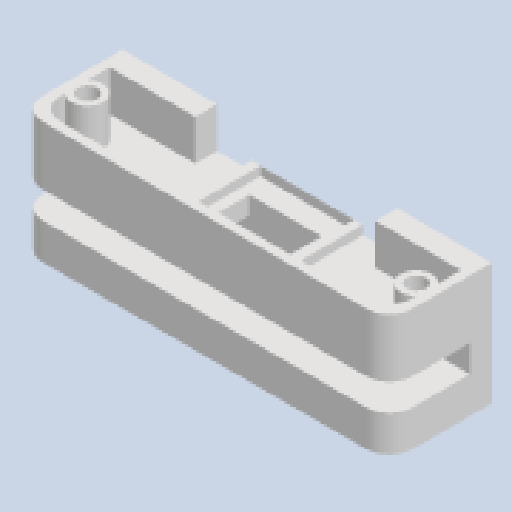
# Autodesk Inventor part: basepcb
Saved by Autodesk Inventor 2026.2 (Build 302298000, 298)
## iProperties
Created: 2026-04-10
Part Number: basepcb
Material: Generic
Document SubType Name: Modeling
Designer: Fork
Density: 1 g/cm^3
Appearance: Default
Author: Fork
Autodesk Inventor part; units mm, degrees
ref_plane "YZ Plane" through (0, 0, 0) normal (1, 0, 0) x (0, 1, 0)
ref_plane "XZ Plane" through (0, 0, 0) normal (0, 1, 0) x (-1, 0, 0)
ref_plane "XY Plane" through (0, 0, 0) normal (0, 0, 1) x (1, 0, 0)
sketch "Sketch1" plane through (0, 0, 0) normal (0, 1, 0) x (-1, 0, 0)
  line L0 (-33.5, 62.1) -> (33.5, 62.1)
  line L1 (33.5, 62.1) -> (33.5, -62.1)
  line L2 (33.5, -62.1) -> (-33.5, -62.1)
  line L3 (-33.5, -62.1) -> (-33.5, 62.1)
  line L4 (-33.5, 62.1) -> (33.5, -62.1) construction
  line L5 (33.5, 62.1) -> (-33.5, -62.1) construction
  line L6 (30.5, -59.1) -> (30.5, 59.1)
  line L7 (30.5, 59.1) -> (-30.5, 59.1)
  line L8 (-30.5, 59.1) -> (-30.5, -59.1)
  line L9 (-30.5, -59.1) -> (30.5, -59.1)
  circle A0 centre (30.5, 59.1) radius 2.25
  circle A1 centre (-30.5, 59.1) radius 2.25
  circle A2 centre (-30.5, -59.1) radius 2.25
  circle A3 centre (30.5, -59.1) radius 2.25
  line L10 (-41, 71) -> (41, 71)
  line L11 (41, 71) -> (41, -71)
  line L12 (41, -71) -> (-41, -71)
  line L13 (-41, -71) -> (-41, 71)
  line L14 (-41, 71) -> (41, -71) construction
  line L15 (41, 71) -> (-41, -71) construction
  line L16 (12.75, 87.6) -> (-7.75, 87.6)
  line L17 (-7.75, 87.6) -> (-7.75, 67.1)
  line L18 (-7.75, 67.1) -> (12.75, 67.1)
  line L19 (12.75, 67.1) -> (12.75, 87.6)
  line L20 (12.75, 87.6) -> (-7.75, 67.1) construction
  line L21 (-7.75, 87.6) -> (12.75, 67.1) construction
  line L22 (41, 71) -> (-41, 71)
  line L23 (-41, 71) -> (-41, 92)
  line L24 (-41, 92) -> (41, 92)
  line L25 (41, 92) -> (41, 71)
  point P0 (0, 0)
  point P1 (2.5, 77.35)
  point P2 (12.75, 77.35)
  point P3 (-41, 71)
  dimension "d0" = 67
  dimension "d1" = 124.2
  dimension "d2" = 3
  dimension "d3" = 4.5
  dimension "d4" = 4.5
  dimension "d5" = 4.5
  dimension "d6" = 4.5
  dimension "d9" = 82
  dimension "d10" = 142
  dimension "d27" = 20.5
  dimension "d28" = 20.5
  dimension "d29" = 5
  dimension "d30" = 28.25
  dimension "d31" = 82
  dimension "d32" = 21
  constraints: 52 end point, 10 parallel, 7 midpoint, 5 perpendicular, 4 centre point, 4 coincident, 4 horizontal, 3 other
  measures "d0" distance of L1.end L2.end
  measures "d1" distance of L0.end L1.end
  measures "d2" distance between parallel lines of L1 L6
  measures "d3" diameter of A0
  measures "d4" diameter of A1
  measures "d5" diameter of A2
  measures "d6" diameter of A3
  measures "d9" distance of L11.end L12.end
  measures "d10" distance of L10.end L11.end
  measures "d27" distance of L18.end L17.end
  measures "d28" distance of L17.end L16.end
  measures "d29" distance between parallel lines of L0 L18
  measures "d30" distance from line of L11 point (12.75, 77.35)
  measures "d31" distance of L23.end L24.end
  measures "d32" distance of L22.end L23.end
extrude "Extrusion1" add sketch "Sketch1" along normal blind 2 contours L0 L1 L2 L3 | L9 A3 L6 | L6 A3 L9 | A3 L9 A2 L8 A1 L7 A0 L6 | A0 L7 L6 | L6 L7 A0 | A2 L8 L9 | L9 L8 A2 | A1 L8 L7 | L7 L8 A1 | L23 L24 L25 L10 L19 L16 L17 | L10 L17 L18 L19 L11 L12 L13 | L17 L16 L19 L10 | L10 L19 L18 L17
sketch "Sketch3" plane through (0, 2, 0) normal (0, 1, 0) x (1, 0, 0)
  line L0 (33.5, -62.1) -> (-33.5, -62.1)
  line L1 (-33.5, -62.1) -> (-33.5, 62.1)
  line L2 (-33.5, 62.1) -> (33.5, 62.1)
  line L3 (33.5, 62.1) -> (33.5, -62.1)
  line L4 (33.5, -62.1) -> (-33.5, 62.1) construction
  line L5 (-33.5, -62.1) -> (33.5, 62.1) construction
  line L6 (-30.5, -59.1) -> (30.5, -59.1)
  line L7 (30.5, -59.1) -> (30.5, 59.1)
  line L8 (30.5, 59.1) -> (-30.5, 59.1)
  line L9 (-30.5, 59.1) -> (-30.5, -59.1)
  circle A0 centre (-30.5, -59.1) radius 2.25
  circle A1 centre (-30.5, 59.1) radius 2.25
  circle A2 centre (30.5, -59.1) radius 2.25
  circle A3 centre (30.5, 59.1) radius 2.25
  circle A4 centre (-30.5, -59.1) radius 5.25
  circle A5 centre (30.5, -59.1) radius 5.25
  circle A6 centre (-30.5, 59.1) radius 5.25
  circle A7 centre (30.5, 59.1) radius 5.25
  point P0 (0, 0)
  dimension "d11" = 67
  dimension "d12" = 124.2
  dimension "d13" = 3
  dimension "d14" = 4.5
  dimension "d15" = 4.5
  dimension "d16" = 4.5
  dimension "d17" = 4.5
  dimension "d18" = 3
  dimension "d19" = 3
  dimension "d20" = 3
  dimension "d21" = 3
  constraints: 20 end point, 8 centre point, 4 coincident, 4 parallel, 2 midpoint, 2 perpendicular, 1 horizontal, 3 other
  measures "d11" distance of L1.end L2.end
  measures "d12" distance of L0.end L1.end
  measures "d13" distance between parallel lines of L0 L6
  measures "d14" diameter of A0
  measures "d15" diameter of A1
  measures "d16" diameter of A2
  measures "d17" diameter of A3
  measures "d18" radial gap between concentric circles of A0 A4
  measures "d19" radial gap between concentric circles of A2 A5
  measures "d20" radial gap between concentric circles of A1 A6
  measures "d21" radial gap between concentric circles of A3 A7
extrude "Extrusion2" add sketch "Sketch3" along normal blind 15 contours L3 A5 L0 | L0 A5 L6 A2 L7 L3 | A4 L1 L0 | L0 L1 A4 L9 A0 L6 | A5 L7 A2 L6 | A7 L7 A3 L8 L2 L3 | L3 L2 A7 | L6 A0 L9 A4 | A7 L8 A3 L7 | A6 L2 L1 | L1 L2 A6 L8 A1 L9 | L9 A1 L8 A6
sketch "Sketch5" plane through (0, 2, 0) normal (0, 1, 0) x (1, 0, 0)
  line L0 (41, 71) -> (-41, 71) projected
  line L1 (-41, 71) -> (-41, -92) projected
  line L2 (41, 71) -> (-41, 71)
  line L3 (-41, 71) -> (-41, -92)
  line L4 (41, -92) -> (41, 71) projected
  line L5 (-41, -66.1) -> (-41, 71)
  circle A0 centre (-30.5, -59.1) radius 5.25 projected
  line L6 (-41, 71) -> (41, 71)
  line L7 (41, 71) -> (41, -71.1)
  line L8 (41, -71.1) -> (-41, -71.1)
  line L9 (-41, -71.1) -> (-41, 71)
  line L10 (-39, -69.1) -> (39, -69.1)
  line L11 (39, -69.1) -> (39, 69)
  line L12 (39, 69) -> (-39, 69)
  line L13 (-39, 69) -> (-39, -69.1)
  line L14 (-20, -69.1) -> (20, -69.1)
  line L15 (20, -69.1) -> (20, -71.1)
  line L16 (20, -71.1) -> (-20, -71.1)
  line L17 (-20, -71.1) -> (-20, -69.1)
  point P0 (0, 0)
  point P1 (-20, -70.1)
  point P2 (0, -69.1)
  point P3 (-41, -71.1)
  dimension "d107" = 12
  dimension "d108" = 2
  dimension "d109" = 2
  dimension "d110" = 2
  dimension "d111" = 2
  dimension "d112" = 40
  dimension "d113" = 2
  dimension "d114" = 20
  constraints: 30 end point, 6 parallel, 4 horizontal, 4 perpendicular, 2 midpoint, 2 point on line
  measures "d107" distance from line of L8 A0.centre
  measures "d108" distance between parallel lines of L1 L13
  measures "d109" distance between parallel lines of L8 L10
  measures "d110" distance between parallel lines of L4 L11
  measures "d111" distance between parallel lines of L0 L12
  measures "d112" distance of L15.end L16.end
  measures "d113" distance of L14.end L15.end
  measures "d114" horizontal distance of point (-20, -70.1) point (0, -69.1)
extrude "Extrusion4" add sketch "Sketch5" along normal blind 25 contours L4 L8 L15 L10 L11 L12 L13 L17 L1 L0
sketch "Sketch7" plane through (0, 2, 0) normal (0, 1, 0) x (1, 0, 0)
  circle A0 centre (-36, 66) radius 2.1
  circle A1 centre (-36, 66) radius 4
  circle A2 centre (36, 66) radius 2.1
  circle A3 centre (-36, -66.1) radius 2.1
  circle A4 centre (36, -66.1) radius 2.1
  circle A5 centre (36, 66) radius 4
  circle A6 centre (36, -66.1) radius 4
  circle A7 centre (-36, -66.1) radius 4
  line L0 (-39, -69.1) -> (-39, 69) projected
  line L1 (-39, 69) -> (39, 69) projected
  line L2 (-20, -69.1) -> (-39, -69.1) projected
  line L3 (39, 69) -> (39, -69.1) projected
  line L4 (39, -69.1) -> (20, -69.1) projected
  point P0 (0, 0)
  dimension "d36" = 4.2
  dimension "d39" = 8
  dimension "d44" = 4.2
  dimension "d45" = 4.2
  dimension "d46" = 4.2
  dimension "d53" = 8
  dimension "d54" = 8
  dimension "d55" = 8
  dimension "d115" = 3
  dimension "d116" = 3
  dimension "d117" = 3
  dimension "d118" = 3
  dimension "d119" = 3
  dimension "d121" = 3
  dimension "d122" = 3
  dimension "d123" = 3
  constraints: 8 centre point, 4 coincident
  measures "d36" diameter of A0
  measures "d39" diameter of A1
  measures "d44" diameter of A2
  measures "d45" diameter of A3
  measures "d46" diameter of A4
  measures "d53" diameter of A5
  measures "d54" diameter of A6
  measures "d55" diameter of A7
  measures "d115" distance from line of L0 A0.centre
  measures "d116" distance from line of L1 A0.centre
  measures "d117" distance from line of L2 A7.centre
  measures "d118" distance from line of L0 A7.centre
  measures "d119" distance from line of L3 A6.centre
  measures "d121" distance from line of L3 A5.centre
  measures "d122" distance from line of L1 A2.centre
  measures "d123" distance from line of L4 A4.centre
extrude "Extrusion5" add sketch "Sketch7" along normal up to surface (25 mm away) contours A1 L0 L1 | L1 A1 | A1 L0 | A5 L3 | L3 A5 L1 | L1 A5 | A6 L3 | L3 A6 L4 | L4 A6 | A7 L2 L0 | L0 A7 | A7 L2 picked at (-35.9156, 68.6949) picked at (36.0844, 68.6949) picked at (36.0844, -68.7949) picked at (-36.0844, -68.7949)
sketch "Sketch8" plane through (0, 2, 0) normal (0, 1, 0) x (1, 0, 0)
  line L0 (41, -92) -> (41, -71.1) projected
  line L1 (-41, -92) -> (41, -92)
  line L2 (41, -92) -> (41, -71.1)
  line L3 (41, -71.1) -> (-41, -71.1)
  line L4 (-41, -71.1) -> (-41, -92)
  point P0 (0, 0)
  point P1 (37.4215, -69.1)
  constraints: 8 end point, 2 parallel, 1 horizontal, 1 perpendicular
extrude "Extrusion6" add sketch "Sketch8" along normal blind 8
sketch "Sketch18" plane through (20, 27, 71.1) normal (0, 0, 1) x (1, 0, 0)
  line L0 (-61, -27) -> (-61, 0) projected
  line L1 (21, -27) -> (21, 0) projected
  line L2 (-61, 0) -> (21, 0)
  line L3 (21, 0) -> (21, -13)
  line L4 (21, -13) -> (-61, -13)
  line L5 (-61, -13) -> (-61, 0)
  line L6 (-61, -17) -> (21, -17) projected
  line L7 (-61, -13) -> (21, -13)
  line L8 (21, -13) -> (21, -3)
  line L9 (21, -3) -> (-61, -3)
  line L10 (-61, -3) -> (-61, -13)
  point P0 (-20, -27)
  point P1 (21, -3)
  dimension "d124" = 4
  dimension "d125" = 10
  constraints: 16 end point, 4 parallel, 2 horizontal, 2 perpendicular, 2 point on line
  measures "d124" distance between parallel lines of L4 L6
  measures "d125" distance of L8.end L7.end
extrude "Extrusion16" add sketch "Sketch18" along normal up to surface (20.9 mm away) contours L0 L9 L1 L4
sketch "Sketch19" plane through (-20, 24, 71.1) normal (0, 1, 0) x (1, 0, 0)
  line L0 (-21, 142.1) -> (-21, -20.9) projected
  line L1 (40, 0) -> (61, 0) projected
  line L2 (-21, -20.9) -> (61, -20.9)
  line L3 (61, -20.9) -> (61, 0)
  line L4 (61, 0) -> (-21, 0)
  line L5 (-21, 0) -> (-21, -20.9)
  line L6 (-19, -2) -> (59, -2)
  line L7 (59, -2) -> (59, -18.9)
  line L8 (59, -18.9) -> (-19, -18.9)
  line L9 (-19, -18.9) -> (-19, -2)
  line L10 (0, 0) -> (0, -2)
  line L11 (40, 0) -> (40, -2)
  point P0 (20, 71.1)
  dimension "d128" = 2
  constraints: 20 end point, 4 parallel, 4 perpendicular, 2 point on line, 1 horizontal, 3 other
  measures "d128" distance between parallel lines of L4 L6
extrude "Extrusion17" cut sketch "Sketch19" against normal blind 6 contours L4 L11 L6 L10 | L6 L7 L8 L9
sketch "Sketch20" plane through (-20, 18, 71.1) normal (0, 1, 0) x (1, 0, 0)
  line L0 (59, -18.9) -> (-19, -18.9) projected
  line L1 (20, -18.9) -> (20, 0)
  line L2 (0, 0) -> (40, 0) projected
  circle A0 centre (12.1, -15.9) radius 1.75
  circle A1 centre (27.9, -15.9) radius 1.75
  point P0 (20, 71.1)
  dimension "d131" = 3.5
  dimension "d132" = 3.5
  dimension "d133" = 15.8
  dimension "d134" = 7.9
  dimension "d135" = 3
  dimension "d136" = 3
  constraints: 2 centre point, 2 end point, 2 midpoint
  measures "d131" diameter of A0
  measures "d132" diameter of A1
  measures "d133" distance of A1.centre A0.centre
  measures "d134" distance from line of A0.centre L1
  measures "d135" distance from line of L0 A0.centre
  measures "d136" distance from line of L0 A1.centre
sketch "Sketch21" plane through (0, 2, 0) normal (0, 1, 0) x (1, 0, 0)
  line L0 (20, -69.1) -> (20, -71.1) projected
  line L1 (-20, -71.1) -> (20, -71.1) projected
  line L2 (20, -69.1) -> (-20, -69.1)
  line L3 (-20, -69.1) -> (-20, -71.1)
  line L4 (-20, -71.1) -> (20, -71.1)
  line L5 (20, -71.1) -> (20, -69.1)
  point P0 (0, 0)
  constraints: 8 end point, 2 parallel, 1 horizontal, 1 perpendicular
extrude "Extrusion18" add sketch "Sketch21" along normal up to surface (16 mm away)
extrude "Extrusion19" cut sketch "Sketch20" against normal blind 4
sketch "Sketch22" plane through (-20, 18, 71.1) normal (0, 1, 0) x (1, 0, 0)
  line L0 (30.35, 1.8) -> (9.65, 1.8)
  line L1 (9.65, 1.8) -> (9.65, -18.9)
  line L2 (9.65, -18.9) -> (30.35, -18.9)
  line L3 (30.35, -18.9) -> (30.35, 1.8)
  line L4 (30.35, 1.8) -> (9.65, -18.9) construction
  line L5 (9.65, 1.8) -> (30.35, -18.9) construction
  line L6 (40, 2) -> (0, 2) projected
  line L7 (20, 2) -> (20, -18.9)
  line L8 (59, -18.9) -> (-19, -18.9) projected
  line L9 (59, -18.9) -> (-19, -18.9) projected
  line L10 (32.35, 3.8) -> (7.65, 3.8)
  line L11 (7.65, 3.8) -> (7.65, -20.9)
  line L12 (7.65, -20.9) -> (32.35, -20.9)
  line L13 (32.35, -20.9) -> (32.35, 3.8)
  point P0 (20, 71.1)
  point P1 (20, -8.55)
  point P2 (20, -18.9)
  point P3 (32.35, -18.9)
  point P4 (32.35, 2)
  point P5 (7.65, 2)
  point P6 (7.65, -18.9)
  point P7 (9.65, -18.9)
  point P8 (30.35, -18.9)
  dimension "d141" = 20.7
  dimension "d142" = 20.7
  dimension "d143" = 0
  dimension "d144" = 0
  dimension "d145" = 2
  constraints: 22 end point, 5 midpoint, 4 parallel, 2 perpendicular, 1 horizontal, 3 other
  measures "d141" distance of L2.end L1.end
  measures "d142" distance of L0.end L1.end
  measures "d143" horizontal distance of point (20, -18.9) point (20, -8.55)
  measures "d144" distance between parallel lines of L8 L2
  measures "d145" distance between parallel lines of L3 L13
extrude "Extrusion20" add sketch "Sketch22" along normal blind 2 contours L0 L7 L6 L13 L8 L3 | L0 L1 L8 L11 L6 L7
sketch "Sketch23" plane through (-20, 18, 71.1) normal (0, 1, 0) x (1, 0, 0)
  line L0 (-13.3542, 2) -> (53.3542, 2) projected
  line L1 (20, 2) -> (20, -18.9)
  line L2 (30.35, -18.9) -> (9.65, -18.9) projected
  line L3 (28, -13.9) -> (12, -13.9)
  line L4 (12, -13.9) -> (12, -1.9)
  line L5 (12, -1.9) -> (28, -1.9)
  line L6 (28, -1.9) -> (28, -13.9)
  circle A0 centre (27.9, -15.9) radius 1.75 projected
  point P0 (20, 71.1)
  point P1 (28, -7.9)
  point P2 (20, -13.9)
  dimension "d148" = 8
  dimension "d149" = 8
  dimension "d150" = 2
  dimension "d151" = 12
  constraints: 10 end point, 4 midpoint, 2 parallel, 1 horizontal, 1 perpendicular
  measures "d148" distance from line of point (28, -7.9) L1
  measures "d149" distance between parallel lines of L4 L1
  measures "d150" vertical distance of A0.centre point (20, -13.9)
  measures "d151" distance between parallel lines of L3 L5
extrude "Extrusion21" cut sketch "Sketch23" against normal blind 4 contours L5 L6 L3 L1 | L1 L3 L4 L5
sketch "Sketch24" plane through (41, 0, -71) normal (0, 0, -1) x (-1, 0, 0)
  line L0 (34.3117, 23.869) -> (40.9117, 23.869) projected
  arc A0 (42.2117, 22.569) -> (40.9117, 23.869) centre (40.9117, 22.569) ccw projected
  line L1 (42.2117, 22.569) -> (42.2117, 21.9283) projected
  line L2 (37.3524, 20.6283) -> (34.3117, 20.6283) projected
  arc A1 (33.0117, 21.9283) -> (34.3117, 20.6283) centre (34.3117, 21.9283) ccw projected
  line L3 (33.0117, 22.3283) -> (33.0117, 21.9283) projected
  arc A2 (34.3117, 23.869) -> (33.0117, 22.569) centre (34.3117, 22.569) ccw projected
  line L4 (33.0117, 21.9283) -> (33.0117, 22.569) projected
  arc A3 (40.9117, 20.6283) -> (42.2117, 21.9283) centre (40.9117, 21.9283) ccw projected
  line L5 (40.9117, 20.6283) -> (37.371, 20.6283) projected
  line L6 (37.371, 20.6283) -> (37.3524, 20.6283) projected
  line L7 (40.9117, 24.169) -> (34.3117, 24.169)
  arc A4 (34.3117, 24.169) -> (32.7117, 22.569) centre (34.3117, 22.569) ccw
  line L8 (32.7117, 22.569) -> (32.7117, 21.9283)
  arc A5 (32.7117, 21.9283) -> (34.3117, 20.3283) centre (34.3117, 21.9283) ccw
  line L9 (34.3117, 20.3283) -> (37.3524, 20.3283)
  line L10 (37.3524, 20.3283) -> (37.371, 20.3283)
  line L11 (37.371, 20.3283) -> (40.9117, 20.3283)
  arc A6 (40.9117, 20.3283) -> (42.5117, 21.9283) centre (40.9117, 21.9283) ccw
  line L12 (42.5117, 21.9283) -> (42.5117, 22.569)
  arc A7 (42.5117, 22.569) -> (40.9117, 24.169) centre (40.9117, 22.569) ccw
  point P0 (41, 0)
  dimension "d154" = 0.3
  constraints: 12 end point, 8 point on circle, 4 centre point, 9 other
  measures "d154" radial gap between concentric circles of A0 A7
extrude "Extrusion22" cut sketch "Sketch24" against normal blind 2 contours L0 A0 L1 A3 L5 L6 L2 A1 L3 L4 A2 | A7 L12 A6 L11 L10 L9 A5 L8 A4 L7
sketch "Sketch25" plane through (-33.3542, 2, -69) normal (0, 0, 1) x (1, 0, 0)
  line L0 (41.6426, 20.569) -> (41.6426, 19.9283) projected
  arc A0 (40.0426, 18.3283) -> (41.6426, 19.9283) centre (40.0426, 19.9283) ccw projected
  line L1 (40.0426, 18.3283) -> (33.4426, 18.3283) projected
  arc A1 (31.8426, 19.9283) -> (33.4426, 18.3283) centre (33.4426, 19.9283) ccw projected
  line L2 (31.8426, 19.9283) -> (31.8426, 20.569) projected
  arc A2 (33.4426, 22.169) -> (31.8426, 20.569) centre (33.4426, 20.569) ccw projected
  line L3 (33.4426, 22.169) -> (40.0426, 22.169) projected
  arc A3 (41.6426, 20.569) -> (40.0426, 22.169) centre (40.0426, 20.569) ccw projected
  line L4 (66.7085, 0) -> (66.7085, 25) projected
  line L5 (0, 25) -> (66.7085, 25) projected
  line L6 (0, 25) -> (0, 0) projected
  line L7 (66.7085, 0) -> (0, 0) projected
  line L8 (30.8426, 20.569) -> (30.8426, 19.9283)
  arc A4 (30.8426, 19.9283) -> (33.4426, 17.3283) centre (33.4426, 19.9283) ccw
  line L9 (33.4426, 17.3283) -> (40.0426, 17.3283)
  arc A5 (40.0426, 17.3283) -> (42.6426, 19.9283) centre (40.0426, 19.9283) ccw
  line L10 (42.6426, 19.9283) -> (42.6426, 20.569)
  arc A6 (42.6426, 20.569) -> (40.0426, 23.169) centre (40.0426, 20.569) ccw
  line L11 (40.0426, 23.169) -> (33.4426, 23.169)
  arc A7 (33.4426, 23.169) -> (30.8426, 20.569) centre (33.4426, 20.569) ccw
  point P0 (33.3542, -2)
  dimension "d157" = 1
  constraints: 8 end point, 8 point on circle, 4 centre point, 7 other
  measures "d157" radial gap between concentric circles of A2 A7
extrude "Extrusion23" add sketch "Sketch25" along normal blind 1 contours A7 L11 A6 L10 A5 L9 A4 L8
sketch "Sketch26" plane through (41, 0, -71) normal (0, 0, -1) x (-1, 0, 0)
  line L0 (28.8617, 19.1283) -> (46.3617, 19.1283)
  line L1 (46.3617, 19.1283) -> (46.3617, 17.1283)
  line L2 (46.3617, 17.1283) -> (28.8617, 17.1283)
  line L3 (28.8617, 17.1283) -> (28.8617, 19.1283)
  line L4 (34.3117, 19.3283) -> (40.9117, 19.3283) projected
  point P0 (41, 0)
  point P1 (37.6117, 19.3283)
  point P2 (28.8617, 18.1283)
  dimension "d160" = 0.2
  dimension "d161" = 17.5
  dimension "d162" = 8.75
  dimension "d163" = 2
  constraints: 8 end point, 2 midpoint, 2 parallel, 1 horizontal, 1 perpendicular
  measures "d160" distance between parallel lines of L4 L0
  measures "d161" distance of L1.end L2.end
  measures "d162" horizontal distance of point (37.612, 19.328) point (28.862, 18.128)
  measures "d163" distance of L0.end L1.end
extrude "Extrusion24" add sketch "Sketch26" against normal blind 8
fillet "Fillet1" radius 5 6 edges at (-41, 13.5, -71) (41, 13.5, -71) (-41, 5, 92) (-41, 19, 92) (41, 5, 92) (41, 19, 92)
sketch "Sketch27" plane through (-41, 10, 71.1) normal (-1, 0, 0) x (0, 0, 1)
  line L0 (-117.1, 11) -> (-109.6, 11)
  line L1 (-109.6, 11) -> (-109.6, 6)
  line L2 (-109.6, 6) -> (-117.1, 6)
  line L3 (-117.1, 6) -> (-117.1, 11)
  line L4 (-142.1, 17) -> (-142.1, -10) projected
  line L5 (-137.1, 17) -> (0, 17) projected
  point P0 (-71.1, -10)
  point P1 (-117.1, 8.5)
  dimension "d167" = 7.5
  dimension "d168" = 5
  dimension "d169" = 25
  dimension "d170" = 6
  constraints: 8 end point, 2 parallel, 1 horizontal, 1 midpoint, 1 perpendicular
  measures "d167" distance of L1.end L2.end
  measures "d168" distance of L0.end L1.end
  measures "d169" distance from line of L4 point (-117.1, 8.5)
  measures "d170" distance between parallel lines of L5 L0
extrude "Extrusion25" cut sketch "Sketch27" against normal blind 2
sketch "Sketch28" plane through (-39, 2, 63.4542) normal (1, 0, 0) x (0, 0, -1)
  line L0 (101.9542, 19) -> (109.4542, 19) projected
  line L1 (101.9542, 14) -> (101.9542, 19) projected
  line L2 (109.4542, 19) -> (101.9542, 19)
  line L3 (101.9542, 19) -> (101.9542, 14)
  line L4 (101.9542, 14) -> (109.4542, 14)
  line L5 (109.4542, 14) -> (109.4542, 19)
  line L6 (110.9542, 13.5) -> (100.4542, 13.5)
  line L7 (100.4542, 13.5) -> (100.4542, 19.5)
  line L8 (100.4542, 19.5) -> (110.9542, 19.5)
  line L9 (110.9542, 19.5) -> (110.9542, 13.5)
  line L10 (110.9542, 13.5) -> (100.4542, 19.5) construction
  line L11 (100.4542, 13.5) -> (110.9542, 19.5) construction
  line L12 (109.4542, 14) -> (109.4542, 19) projected
  line L13 (115.7042, 13.5) -> (95.7042, 13.5)
  line L14 (95.7042, 13.5) -> (95.7042, 19.5)
  line L15 (95.7042, 19.5) -> (115.7042, 19.5)
  line L16 (115.7042, 19.5) -> (115.7042, 13.5)
  line L17 (115.7042, 13.5) -> (95.7042, 19.5) construction
  line L18 (95.7042, 13.5) -> (115.7042, 19.5) construction
  line L19 (115.7042, 13.5) -> (111.7042, 13.5)
  line L20 (111.7042, 13.5) -> (111.7042, 12.5)
  line L21 (111.7042, 12.5) -> (115.7042, 12.5)
  line L22 (115.7042, 12.5) -> (115.7042, 13.5)
  line L23 (95.7042, 13.5) -> (99.7042, 13.5)
  line L24 (99.7042, 13.5) -> (99.7042, 12.5)
  line L25 (99.7042, 12.5) -> (95.7042, 12.5)
  line L26 (95.7042, 12.5) -> (95.7042, 13.5)
  point P0 (63.4542, -2)
  point P1 (105.7042, 16.5)
  point P2 (105.7042, 19.5)
  point P3 (110.9542, 16.5)
  point P4 (109.4542, 16.5)
  dimension "d173" = 10.5
  dimension "d174" = 6
  dimension "d175" = 0.5
  dimension "d176" = 1.5
  dimension "d177" = 20
  dimension "d178" = 4
  dimension "d179" = 1
  dimension "d180" = 4
  dimension "d181" = 1
  constraints: 48 end point, 10 parallel, 7 midpoint, 5 horizontal, 5 perpendicular, 1 point on line
  measures "d173" distance of L7.end L8.end
  measures "d174" distance of L6.end L7.end
  measures "d175" distance from line of point (105.704, 19.5) L0
  measures "d176" distance of point (110.954, 16.5) point (109.454, 16.5)
  measures "d177" distance of L14.end L15.end
  measures "d178" distance of L21.end L20.end
  measures "d179" distance of L20.end L19.end
  measures "d180" distance of L24.end L25.end
  measures "d181" distance of L23.end L24.end
extrude "Extrusion26" add sketch "Sketch28" along normal blind 1 contours L13 L22 L21 L20 | L24 L25 L26 L13
sketch "Sketch29" plane through (-38, 2, 63.4542) normal (1, 0, 0) x (0, 0, -1)
  line L0 (111.7042, 12.5) -> (111.7042, 13.5) projected
  line L1 (115.7042, 12.5) -> (111.7042, 12.5)
  line L2 (111.7042, 12.5) -> (111.7042, 13.5)
  line L3 (111.7042, 13.5) -> (115.7042, 13.5)
  line L4 (115.7042, 13.5) -> (115.7042, 12.5)
  line L5 (99.7042, 12.5) -> (99.7042, 13.5) projected
  line L6 (95.7042, 12.5) -> (95.7042, 13.5) projected
  line L7 (99.7042, 12.5) -> (95.7042, 12.5)
  line L8 (95.7042, 12.5) -> (95.7042, 13.5)
  line L9 (95.7042, 13.5) -> (99.7042, 13.5)
  line L10 (99.7042, 13.5) -> (99.7042, 12.5)
  line L11 (115.7042, 12.5) -> (111.7042, 12.5)
  line L12 (111.7042, 12.5) -> (111.7042, 17.5)
  line L13 (111.7042, 17.5) -> (115.7042, 17.5)
  line L14 (115.7042, 17.5) -> (115.7042, 12.5)
  line L15 (99.7042, 12.5) -> (95.7042, 12.5)
  line L16 (95.7042, 12.5) -> (95.7042, 17.5)
  line L17 (95.7042, 17.5) -> (99.7042, 17.5)
  line L18 (99.7042, 17.5) -> (99.7042, 12.5)
  point P0 (63.4542, -2)
  dimension "d184" = 5
  dimension "d185" = 5
  constraints: 32 end point, 8 parallel, 4 horizontal, 4 perpendicular, 2 point on line
  measures "d184" distance of L11.end L12.end
  measures "d185" distance of L15.end L16.end
extrude "Extrusion27" add sketch "Sketch29" along normal blind 1
chamfer "Chamfer1" distance 2 angle 45 2 edges at (-39, 14.5, -34.25) (-39, 14.5, -50.25)
sketch "Sketch30" plane through (20, 24, 71.1) normal (0, 1, 0) x (1, 0, 0)
  arc A0 (16, -20.9) -> (21, -15.9) centre (16, -15.9) ccw projected
  line L0 (21, 0) -> (21, -15.9) projected
  line L1 (0, 0) -> (21, 0) projected
  line L2 (0, 0) -> (0, -2) projected
  line L3 (0, -2) -> (19, -2) projected
  line L4 (19, -2) -> (19, -18.9) projected
  line L5 (19, -18.9) -> (-59, -18.9) projected
  line L6 (-59, -18.9) -> (-59, -2) projected
  line L7 (-59, -2) -> (-40, -2) projected
  line L8 (-40, -2) -> (-40, 0) projected
  line L9 (-61, 0) -> (-40, 0) projected
  line L10 (-61, 0) -> (-61, -15.9) projected
  arc A1 (-61, -15.9) -> (-56, -20.9) centre (-56, -15.9) ccw projected
  line L11 (-56, -20.9) -> (16, -20.9) projected
  point P0 (-20, 71.1)
extrude "Extrusion28" add sketch "Sketch30" along normal up to surface (3 mm away)
fillet "Fillet2" radius 5 2 edges at (-39, 22.5, 90) (39, 22.5, 90)
sketch "Sketch33" plane through (-20, 18, 71.1) normal (0, 1, 0) x (1, 0, 0)
  arc A0 (-19, -13.9) -> (-14, -18.9) centre (-14, -13.9) ccw projected
  line L0 (7.65, -18.9) -> (-14, -18.9) projected
  line L1 (7.65, -18.9) -> (7.65, 2) projected
  line L2 (7.65, 2) -> (0, 2) projected
  line L3 (0, -2) -> (0, 2) projected
  line L4 (-19, -2) -> (0, -2) projected
  line L5 (-19, -13.9) -> (-19, -2) projected
  arc A1 (54, -18.9) -> (59, -13.9) centre (54, -13.9) ccw projected
  line L6 (59, -2) -> (59, -13.9) projected
  line L7 (40, -2) -> (59, -2) projected
  line L8 (40, 2) -> (40, -2) projected
  line L9 (40, 2) -> (32.35, 2) projected
  line L10 (32.35, 2) -> (32.35, -18.9) projected
  line L11 (54, -18.9) -> (32.35, -18.9) projected
  line L12 (-14, -2) -> (-14, -18.9)
  line L13 (-21, 137.1) -> (-21, -15.9) projected
  line L14 (-14, -10.45) -> (-19, -10.45)
  circle A2 centre (-16.5, -10.45) radius 2.1
  circle A3 centre (-16.5, -10.45) radius 3.5
  line L15 (54, -2) -> (54, -18.9)
  line L16 (54, -10.45) -> (59, -10.45)
  circle A4 centre (56.5, -10.45) radius 2.1
  circle A5 centre (56.5, -10.45) radius 3.5
  point P0 (20, 71.1)
  point P1 (59, -8.0005)
  point P2 (59, -12.8995)
  dimension "d198" = 4.2
  dimension "d199" = 7
  dimension "d202" = 4.2
  dimension "d203" = 7
  constraints: 8 end point, 4 centre point, 4 midpoint, 4 point on line, 2 coincident, 2 perpendicular, 1 parallel, 1 vertical
  measures "d198" diameter of A2
  measures "d199" diameter of A3
  measures "d202" diameter of A4
  measures "d203" diameter of A5
extrude "Extrusion30" add sketch "Sketch33" along normal up to surface (9 mm away) contours A3 L5 | L5 L14 A2 L12 A3 | L12 A3 | L5 A3 L12 L14 A2 | A5 L15 | L15 L16 A4 L6 A5 | L15 A5 L6 L16 A4
body "Solid1"
